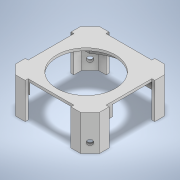
# Autodesk Inventor part: 로드셀 부품2
Saved by Autodesk Inventor 2021 (Build 250183000, 183)
## iProperties
Created: 2021-08-23
Part Number: 로드셀 부품2
Material: 일반
Document SubType Name: Modeling
Designer: Dongyoon
Density: 1 g/cm^3
Appearance: 기본값
Author: Dongyoon
Autodesk Inventor part; units mm, degrees
ref_plane "YZ Plane" through (0, 0, 0) normal (1, 0, 0) x (0, 1, 0)
ref_plane "XZ Plane" through (0, 0, 0) normal (0, 1, 0) x (-1, 0, 0)
ref_plane "XY Plane" through (0, 0, 0) normal (0, 0, 1) x (1, 0, 0)
sketch "스케치1" plane through (0, 0, 0) normal (0, 1, 0) x (-1, 0, 0)
  line L0 (20, 20.5) -> (-20, 20.5)
  line L1 (-20, 20.5) -> (-20, -19.5)
  line L2 (-20, -19.5) -> (20, -19.5)
  line L3 (20, -19.5) -> (20, 20.5)
  line L4 (20, 20.5) -> (-20, -19.5) construction
  line L5 (-20, 20.5) -> (20, -19.5) construction
  circle A0 centre (0, 2.5) radius 15
  point P0 (0, 0)
  dimension "d3" = 40
  dimension "d4" = 40
  dimension "d7" = 30
  dimension "d8" = 22
  dimension "d9" = 20
  dimension "d10" = 2.5
  dimension "d11" = 20
  constraints: 12 end point, 2 parallel, 1 centre point, 1 horizontal, 1 perpendicular
  measures "d3" distance of L1.end L2.end
  measures "d4" distance of L0.end L1.end
  measures "d7" diameter of A0
  measures "d8" distance from line of L2 A0.centre
  measures "d9" distance from line of L1 A0.centre
  measures "d10" distance of point (0, 0) A0.centre
  measures "d11" distance from line of L1 point (0, 0)
extrude "돌출1" add sketch "스케치1" along normal blind 1.3
sketch "스케치2" plane through (0, 0, 0) normal (0, -1, 0) x (1, 0, 0)
  line L0 (20, 20.5) -> (20, -19.5) projected
  line L1 (20, -15.2) -> (15.7, -19.5)
  line L2 (20, -19.5) -> (-20, -19.5) projected
  line L3 (-15.7, -19.5) -> (-20, -15.2)
  line L4 (-20, -19.5) -> (-20, 20.5) projected
  line L5 (-20, 16.2) -> (-15.7, 20.5)
  line L6 (-20, 20.5) -> (20, 20.5) projected
  line L7 (15.7, 20.5) -> (20, 16.2)
  line L8 (-16.7456, -21) -> (-21.5, -16.2456)
  line L9 (15.7, 20.5) -> (-15.7, 20.5)
  line L10 (-20, 16.2) -> (-20, -15.2)
  line L11 (-15.7, -19.5) -> (15.7, -19.5)
  line L12 (20, -15.2) -> (20, 16.2)
  line L13 (-21.5, -16.2456) -> (-21.5, -11.2456)
  line L14 (-16.7456, -21) -> (-11.7456, -21)
  line L15 (-21.5, -11.2456) -> (-20, -11.2456)
  line L16 (-11.7456, -21) -> (-11.7456, -19.5)
  line L17 (0, -19.5) -> (0, 20.5)
  line L18 (20, 0.5) -> (-20, 0.5)
  line L19 (16.7456, -21) -> (21.5, -16.2456)
  line L20 (21.5, -16.2456) -> (21.5, -11.2456)
  line L21 (16.7456, -21) -> (11.7456, -21)
  line L22 (21.5, -11.2456) -> (20, -11.2456)
  line L23 (11.7456, -21) -> (11.7456, -19.5)
  line L24 (-16.7456, 22) -> (-21.5, 17.2456)
  line L25 (-21.5, 17.2456) -> (-21.5, 12.2456)
  line L26 (-16.7456, 22) -> (-11.7456, 22)
  line L27 (-21.5, 12.2456) -> (-20, 12.2456)
  line L28 (-11.7456, 22) -> (-11.7456, 20.5)
  line L29 (11.7456, 22) -> (11.7456, 20.5)
  line L30 (16.7456, 22) -> (11.7456, 22)
  line L31 (16.7456, 22) -> (21.5, 17.2456)
  line L32 (21.5, 17.2456) -> (21.5, 12.2456)
  line L33 (21.5, 12.2456) -> (20, 12.2456)
  point P0 (0, 0)
  point P1 (20, -11.2456)
  point P2 (11.7456, -19.5)
  point P3 (11.7456, 20.5)
  point P4 (20, 12.2456)
  point P5 (-20, 12.2456)
  point P6 (-11.7456, 20.5)
  point P7 (-11.7456, -19.5)
  point P8 (-20, -11.2456)
  point P9 (18.2456, 20.5)
  point P10 (20, 18.7456)
  point P11 (-20, 18.7456)
  point P12 (-18.2456, 20.5)
  point P13 (-18.2456, -19.5)
  point P14 (-20, -17.7456)
  point P15 (20, -17.7456)
  point P16 (18.2456, -19.5)
  dimension "d15" = 4.3
  dimension "d16" = 4.3
  dimension "d17" = 4.3
  dimension "d18" = 4.3
  dimension "d19" = 4.3
  dimension "d20" = 4.3
  dimension "d21" = 1.8
  dimension "d25" = 5
  dimension "d26" = 5
  dimension "d28" = 1.5
  dimension "d29" = 1.5
  constraints: 60 end point, 18 symmetric about line, 10 point on line, 4 midpoint, 4 perpendicular, 3 collinear, 2 horizontal, 2 parallel
  measures "d15" distance of L2.end L3.start
  measures "d16" distance of L2.end L3.end
  measures "d17" distance of L0.end L1.start
  measures "d18" distance of L4.end L5.start
  measures "d19" distance of L4.end L5.end
  measures "d20" distance of L0.start L7.end
  measures "d21" distance between parallel lines of L3 L8
  measures "d25" distance of L8.end L13.end
  measures "d26" distance of L8.start L14.end
  measures "d28" distance of L13.end L15.end
  measures "d29" distance of L14.end L16.end
extrude "돌출2" add sketch "스케치2" along normal blind 17 and the other way blind 1.3 contours L0 L31 L32 L33 | L7 L6 L31 L0 | L6 L29 L30 L31 | L22 L20 L19 L0 | L0 L19 L2 L1 | L6 L24 L26 L28 | L2 L19 L21 L23 | L16 L14 L8 L2 | L4 L8 L13 L15 | L27 L25 L24 L4 | L5 L4 L24 L6 | L2 L8 L4 L3
extrude "돌출3" cut sketch "스케치2" against normal blind 1.5 contours L31 L6 L0 | L0 L2 L19 | L24 L4 L6 | L2 L4 L8
sketch "스케치8" plane through (0, 0, 0) normal (0, -1, 0) x (1, 0, 0)
  circle A0 centre (0, 2.5) radius 15 projected
  circle A1 centre (0, 2.5) radius 21
  line L0 (15.7, -19.5) -> (11.7456, -19.5) projected
  line L1 (-20, -15.2) -> (-15.7, -19.5) projected
  line L2 (15.7, -19.5) -> (-15.7, -19.5)
  line L3 (-15.7, -19.5) -> (-20, -15.2)
  line L4 (-20, -15.2) -> (-20, -3.9031)
  line L5 (-20, -11.2456) -> (-20, 12.2456) projected
  line L6 (15.7, -19.5) -> (20, -15.2) projected
  line L7 (15.7, -19.5) -> (20, -15.2)
  line L8 (20, -15.2) -> (20, -3.9031)
  line L9 (20, 12.2456) -> (20, -11.2456) projected
  line L10 (20, 16.2) -> (15.7, 20.5) projected
  line L11 (20, 16.2) -> (20, 8.9031)
  line L12 (11.7456, 20.5) -> (15.7, 20.5) projected
  line L13 (20, 16.2) -> (15.7, 20.5)
  line L14 (15.7, 20.5) -> (10.8167, 20.5)
  line L15 (-11.7456, 20.5) -> (11.7456, 20.5) projected
  line L16 (-15.7, 20.5) -> (-11.7456, 20.5) projected
  line L17 (-15.7, 20.5) -> (-10.8167, 20.5)
  line L18 (-15.7, 20.5) -> (-20, 16.2) projected
  line L19 (-15.7, 20.5) -> (-20, 16.2)
  line L20 (-20, 16.2) -> (-20, 8.9031)
  line L21 (-20, -15.2) -> (-20, -11.2456) projected
  line L22 (-20, -13.2228) -> (13.921, -13.2228)
  line L23 (13.921, -13.2228) -> (20, -13.2228)
  line L24 (20, -11.2456) -> (20, -15.2) projected
  point P0 (0, 0)
  point P1 (20, 8.9031)
  point P2 (-20, 12.2456)
  point P3 (-20, 8.9031)
  point P4 (-10.8167, 20.5)
  point P5 (-13.921, -13.2228)
  dimension "d45" = 42
  constraints: 26 end point, 6 point on line, 3 collinear, 2 midpoint, 2 perpendicular, 1 coincident, 1 horizontal, 9 other
extrude "돌출6" add sketch "스케치8" along normal blind 5.5 contours A1 L14 L12 L10 L11 L9 | L23 L8 L6 L0 L2 L1 L4 L22 A1 | A1 L5 L20 L18 L16 L15
sketch "스케치9" plane through (-16.7456, -17, -21) normal (-0.7071, 0, -0.7071) x (-0.7071, 0, 0.7071)
  line L0 (-10.2239, 18.3) -> (19.7761, 18.3) projected
  circle A0 centre (3.3619, 5) radius 1.4
  line L1 (6.7238, 0) -> (0, 0) projected
  line L2 (3.3619, 0) -> (3.3619, 21.9108)
  point P0 (3.0083, 17)
  dimension "d48" = 2.8
  dimension "d49" = 5
  constraints: 2 end point, 1 centre point, 1 midpoint, 1 point on line, 1 vertical
  measures "d48" diameter of A0
  measures "d49" distance from line of L1 A0.centre
extrude "돌출7" cut sketch "스케치9" against normal through all
mirror "미러2" about plane through (0, 0, 0) normal (1, 0, 0) of "돌출7"
sketch "스케치10" plane through (0, 0, 0) normal (0, -1, 0) x (1, 0, 0)
  line L0 (0.65, -19.5) -> (-0.65, -19.5)
  line L1 (-0.65, -19.5) -> (-0.65, -17.5)
  line L2 (-0.65, -17.5) -> (0.65, -17.5)
  line L3 (0.65, -17.5) -> (0.65, -19.5)
  arc A0 (-13.921, -13.2228) -> (13.921, -13.2228) centre (0, 2.5) ccw projected
  line L4 (0.65, -19.5) -> (-0.65, -17.5) construction
  line L5 (-0.65, -19.5) -> (0.65, -17.5) construction
  point P0 (0, 0)
  point P1 (0, -18.5)
  dimension "d53" = 1.3
  dimension "d54" = 1
  constraints: 12 end point, 2 midpoint, 2 parallel, 1 horizontal, 1 perpendicular, 1 point on circle
  measures "d53" distance of L1.end L2.end
  measures "d54" vertical distance of point (0, -18.5) L1.end
extrude "돌출8" add sketch "스케치10" along normal blind 5.5
